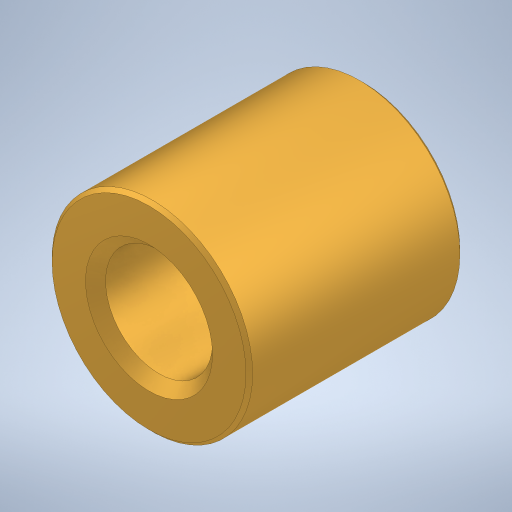
# Autodesk Inventor part: Regular Bushing
Saved by Autodesk Inventor 2023 (Build 270158000, 158)
## iProperties
Created: 2023-02-23
Part Number: Regular Bushing
Material: Brass, Soft Yellow
Document SubType Name: Modeling
Designer: EvanA
Density: 8.47 g/cm^3
Appearance: Brass - Satin
Author: EvanA
Autodesk Inventor part; units mm, degrees
ref_plane "YZ Plane" through (0, 0, 0) normal (1, 0, 0) x (0, 1, 0)
ref_plane "XZ Plane" through (0, 0, 0) normal (0, 1, 0) x (-1, 0, 0)
ref_plane "XY Plane" through (0, 0, 0) normal (0, 0, 1) x (1, 0, 0)
sketch "Sketch1" plane through (0, 0, 0) normal (0, 0, 1) x (1, 0, 0)
  circle A0 centre (0, 0) radius 4
  circle A1 centre (0, 0) radius 7.5
  dimension "d0" = 15
  dimension "d1" = 8
  constraints: 2 centre point, 2 coincident
  measures "d0" diameter of A1
  measures "d1" diameter of A0
extrude "Extrusion1" add sketch "Sketch1" along normal blind 16
chamfer "Chamfer1" distance 0.25 angle 45 2 edges at (-7.5, 0, 16) (-7.5, 0, 0)
chamfer "Chamfer2" distance 0.75 angle 45 2 edges at (-4, 0, 16) (-4, 0, 0)
body "Solid1"
